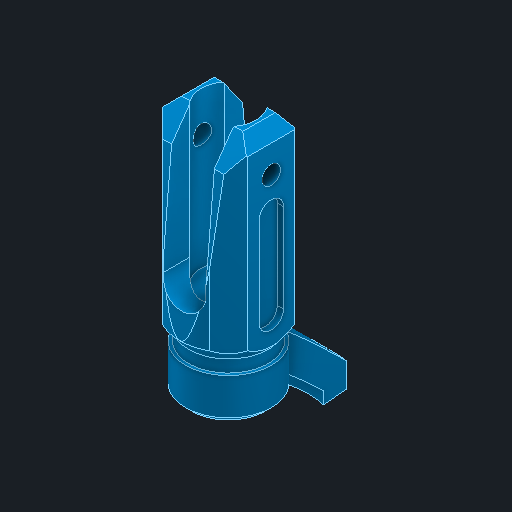
# Autodesk Inventor part: RotorArm
Saved by Autodesk Inventor 2023.2 (Build 272271000, 271)
## iProperties
Created: 2023-03-30
Part Number: RotorArm
Material: Aluminium 6061
Document SubType Name: Modeling
Designer: tadeu
Density: 2.7 g/cm^3
Appearance: Aluminium - flach
Author: tadeu
Autodesk Inventor part; units mm, degrees
ref_plane "YZ Plane" through (0, 0, 0) normal (1, 0, 0) x (0, 1, 0)
ref_plane "XZ Plane" through (0, 0, 0) normal (0, 1, 0) x (-1, 0, 0)
ref_plane "XY Plane" through (0, 0, 0) normal (0, 0, 1) x (1, 0, 0)
sketch "Skizze1" plane through (0, 0, 0) normal (0, 1, 0) x (-1, 0, 0)
  circle A0 centre (0, 0) radius 7
  circle A1 centre (0, 0) radius 6.5
  circle A2 centre (0, 0) radius 2
  dimension "d0" = 14
  dimension "d3" = 13
  dimension "d54" = 4
  constraints: 3 centre point, 3 coincident
  measures "d0" diameter of A0
  measures "d3" diameter of A1
  measures "d54" diameter of A2
extrude "Extrusion1" add sketch "Skizze1" against normal blind 7 contours A0 | A1 | A2
chamfer "Fase1" distance 1 angle 45 1 edges at (7, -7, 0)
extrude "Extrusion2" add sketch "Skizze1" along normal blind 4 contours A1 | A2
sketch "Skizze2" plane through (0, 4, 0) normal (0, 1, 0) x (1, 0, 0)
  circle A0 centre (0, 0) radius 8
  dimension "d9" = 16
  constraints: 1 centre point, 1 coincident
  measures "d9" diameter of A0
extrude "Extrusion3" add sketch "Skizze2" along normal blind 29.5
extrude "Extrusion7" cut sketch "Skizze1" along normal through all both and the other way through all contours A2
chamfer "Fase2" distance 1.5 distance2 2 1 edges at (6.5, 4, 0) measured on face at (7, 4, 0)
sketch "Skizze3" plane through (0, 33.5, 0) normal (0, 1, 0) x (1, 0, 0)
  circle A0 centre (0, 0) radius 8 projected
  line L0 (-7, 3.873) -> (-7, -3.873)
  line L1 (7, -3.873) -> (7, 3.873)
  line L2 (7, 3.873) -> (-7, -3.873) construction
  line L3 (-7, 3.873) -> (7, -3.873) construction
  arc A1 (7, -3.873) -> (7, 3.873) centre (0, 0) ccw
  arc A2 (-7, 3.873) -> (-7, -3.873) centre (0, 0) ccw
  line L4 (7, -3.873) -> (3.873, -7)
  arc A3 (3.873, -7) -> (7, -3.873) centre (0, 0) ccw
  line L5 (7, 3.873) -> (3.873, 7)
  arc A4 (7, 3.873) -> (3.873, 7) centre (0, 0) ccw
  line L6 (0, -7.9724) -> (0, 9.2995) construction
  line L7 (-7, -3.873) -> (-3.873, -7)
  line L8 (-7, -3.873) -> (-3.873, -7)
  line L9 (-7, 3.873) -> (-3.873, 7)
  arc A5 (-3.873, -7) -> (-7, -3.873) centre (0, 0) ccw
  arc A6 (-7, -3.873) -> (-3.873, -7) centre (0, 0) ccw
  arc A7 (-3.873, 7) -> (-7, 3.873) centre (0, 0) ccw
  line L10 (0, 14.4823) -> (0, -23.1738) construction
  point P0 (-4.6045, -6.2685)
  point P1 (-7, 3.873)
  point P2 (-7, 3.873)
  point P3 (6.046, 5.2389)
  point P4 (7, -3.873)
  point P5 (7, -3.873)
  dimension "d15" = 14
  dimension "d26" = 7
  dimension "d33" = 135
  dimension "d34" = 135
  dimension "d35" = 135
  dimension "d36" = 135
  dimension "d48" = 7
  dimension "d49" = 14
  constraints: 22 end point, 16 point on circle, 7 centre point, 2 midpoint, 2 parallel, 2 point on line, 2 vertical, 1 concentric, 13 other
  measures "d15" distance of L1.start L0.end
  measures "d26" distance between parallel lines of L0 L10
  measures "d33" angle of L0 L9
  measures "d34" angle of L7 L0
  measures "d35" angle of L1 L5
  measures "d36" angle of L4 L1
  measures "d48" distance from line of L10 L1.end
  measures "d49" diameter of L0.start L6
extrude "Extrusion4" cut sketch "Skizze3" against normal through all contours A0 L1 | L5 A0 | A0 L4 | L9 A0 | A0 L7 | L0 A0
sketch "Skizze5" plane through (0, 0, 0) normal (0, 0, 1) x (1, 0, 0)
  line L0 (-3.5, 11.5) -> (-3.5, 33.5)
  line L1 (3.873, 33.5) -> (-3.873, 33.5) projected
  line L2 (-7, 33.5) -> (-3.873, 33.5) projected
  line L3 (6.5, 2) -> (-6.5, 2) projected
  line L4 (3.5, 11.5) -> (3.5, 33.5)
  line L5 (-3.5, 33.5) -> (3.5, 33.5)
  line L6 (7, 33.5) -> (3.873, 33.5) projected
  arc A0 (-3.5, 11.5) -> (3.5, 11.5) centre (0, 11.5) ccw
  line L7 (-3.873, 33.5) -> (-3.873, 4) projected
  line L8 (-7, 4) -> (-7, 33.5) projected
  point P0 (0, 0)
  dimension "d28" = 22
  dimension "d29" = 9.5
  dimension "d51" = 7
  constraints: 6 end point, 2 point on circle, 1 centre point, 1 collinear, 1 point on line, 1 vertical
  measures "d28" distance from line of L1 A0.centre
  measures "d29" distance from line of L3 A0.centre
  measures "d51" distance from line of L8 A0.centre
extrude "Extrusion5" cut sketch "Skizze5" along normal through all both and the other way through all
sketch "Skizze6" plane through (0, 0, 0) normal (1, 0, 0) x (0, 1, 0)
  line L0 (4, -8) -> (8, -8) projected
  line L1 (4, -8) -> (29, -5.8128)
  line L2 (4, 8) -> (8, 8) projected
  line L3 (4, -8) -> (4, -7) projected
  line L4 (44.5462, 8) -> (44.5462, -8)
  line L5 (8, -8) -> (44.5462, -8)
  line L6 (8, -8) -> (4, -8)
  line L7 (4, 8) -> (8, 8)
  line L8 (4, 8) -> (29, 5.8128)
  line L9 (4, 8) -> (29.0955, 8) construction
  line L10 (4, 7) -> (4, 8) projected
  line L11 (29, -5.8128) -> (37.3015, 0)
  line L12 (29, -5.8128) -> (39.1343, -5.8128) construction
  line L13 (29, 5.8128) -> (37.3015, 0)
  line L14 (29, 5.8128) -> (39.1343, 5.8128) construction
  line L15 (44.5462, 8) -> (4, 8)
  point P0 (0, 0)
  dimension "d39" = 25
  dimension "d42" = 5
  dimension "d43" = 25
  dimension "d44" = 5
  dimension "d52" = 35
  dimension "d53" = 35
  constraints: 24 end point, 4 horizontal, 3 equal length, 1 collinear, 1 perpendicular, 1 point on line, 1 vertical
  measures "d39" distance from line of L3 L1.end
  measures "d42" angle of L8 L9
  measures "d43" distance from line of L10 L8.end
  measures "d44" angle of L5 L1
  measures "d52" angle of L12 L11
  measures "d53" angle of L13 L14
extrude "Extrusion6" cut sketch "Skizze6" along normal through all both and the other way through all
sketch "Skizze11" plane through (0, 0, 0) normal (1, 0, 0) x (0, 1, 0)
  line L0 (0, -7) -> (-10, -17)
  line L1 (0, -7) -> (21.0348, -7) construction
  line L2 (-6, -7) -> (-12, -13)
  line L3 (-12, -13) -> (-14, -13)
  line L4 (-10, -17) -> (-14, -17)
  line L5 (-14, -13) -> (-14, -17)
  line L6 (42.8428, 0) -> (-25, 0)
  line L7 (0, -7) -> (-6, -7)
  point P0 (0, 0)
  dimension "d64" = 135
  dimension "d67" = 2
  constraints: 16 end point, 4 horizontal, 1 parallel, 1 vertical
  measures "d64" angle of L0 L1
  measures "d67" distance of L2.end L3.end
revolve "Umdrehung2" add sketch "Skizze11" angle 90 mid plane about axis through (0, 42.8428, 0) along (0, -1, 0)
sketch "Skizze16" plane through (0, -7, 0) normal (0, -1, 0) x (1, 0, 0)
  line L0 (0, 0) -> (0, -8.9764) construction
  arc A0 (-4.9497, -4.9497) -> (4.9497, -4.9497) centre (0, 0) ccw construction
  line L1 (12.0208, -12.0208) -> (4.9497, -4.9497) projected
  arc A1 (3.5, -6.0622) -> (4.9497, -4.9497) centre (0, 0) ccw
  arc A2 (2.5, -16.8152) -> (12.0208, -12.0208) centre (0, 0) ccw
  line L2 (2.5, -16.8152) -> (3.5, -6.0622)
  line L3 (9.1924, -9.1924) -> (12.0208, -12.0208) projected
  line L4 (4.9497, -4.9497) -> (12.0208, -12.0208)
  line L5 (-12.0208, -12.0208) -> (-4.9497, -4.9497)
  arc A3 (-4.9497, -4.9497) -> (-3.5, -6.0622) centre (0, 0) ccw
  arc A4 (-12.0208, -12.0208) -> (-2.5, -16.8152) centre (0, 0) ccw
  line L6 (-2.5, -16.8152) -> (-3.5, -6.0622)
  line L7 (-9.1924, -9.1924) -> (-12.0208, -12.0208)
  line L8 (-4.9497, -4.9497) -> (-12.0208, -12.0208)
  dimension "d79" = 3.5
  dimension "d80" = 2.5
  constraints: 14 end point, 9 point on circle, 7 symmetric about line, 4 centre point, 1 collinear, 1 vertical, 2 other
  measures "d79" distance from line of L0 L2.end
  measures "d80" distance from line of L0 L2.start
extrude "Extrusion12" cut sketch "Skizze16" along normal mid plane 14
chamfer "Fase4" distance 2 angle 45 2 edges at (7, 33.5, 0) (-7, 33.5, 0)
sketch "Skizze17" plane through (7, 4, 3.873) normal (1, 0, 0) x (0, 0, -1)
  line L0 (7.746, 0) -> (7.746, 27.5) projected
  line L1 (0, 0) -> (0, 27.5) projected
  line L2 (0, 27.5) -> (7.746, 27.5) projected
  line L3 (10.873, 11.4301) -> (10.873, 0) projected
  line L4 (-3.127, 0) -> (-3.127, 11.4301) projected
  line L5 (6.5348, 29.5) -> (1.2111, 29.5) projected
  point P0 (3.873, -4)
  point P1 (3.873, 23)
  dimension "d100" = 4.5
  dimension "d101" = 7
  dimension "d102" = 14
  dimension "d122" = 2
  measures "d100" distance from line of L2 point (3.873, 23)
  measures "d101" distance from line of point (3.873, 23) L3
  measures "d102" distance between parallel lines of L4 L3
  measures "d122" distance between parallel lines of L5 L2
hole "Bohrung1" at (7, 27, 0) direction (-1, 0, 0) diameter 3 end through all
sketch "Skizze18" plane through (7, 4, 3.873) normal (1, 0, 0) x (0, 0, -1)
  arc A0 (5.873, 17.5) -> (1.873, 17.5) centre (3.873, 17.5) ccw
  line L0 (10.873, 11.4301) -> (10.873, 0) projected
  line L1 (0, 27.5) -> (7.746, 27.5) projected
  arc A1 (1.873, 3) -> (5.873, 3) centre (3.873, 3) ccw
  line L2 (5.873, 17.5) -> (5.873, 3)
  line L3 (1.873, 17.5) -> (1.873, 3)
  point P0 (3.873, -4)
  dimension "d103" = 4
  dimension "d104" = 7
  dimension "d105" = 10
  dimension "d106" = 4
  dimension "d107" = 14.5
  constraints: 4 end point, 4 point on circle, 2 centre point
  measures "d103" diameter of A0
  measures "d104" distance from line of L0 A0.centre
  measures "d105" distance from line of L1 A0.centre
  measures "d106" diameter of A1
  measures "d107" distance of A1.centre A0.centre
extrude "Extrusion13" cut sketch "Skizze18" against normal blind 1
mirror "Spiegeln1" about plane through (0, 0, 0) normal (1, 0, 0) of "Extrusion13"
sketch "Skizze19" plane through (0, -14, 0) normal (0, -1, 0) x (1, 0, 0)
  arc A0 (-2.8849, -12.6758) -> (2.8849, -12.6758) centre (0, 0) ccw projected
  line L0 (0, 0) -> (0, -25.3641) construction
  point P0 (0, 0)
  point P1 (0, -15)
  dimension "d117" = 15
  dimension "d118" = 0
  constraints: 2 end point, 1 vertical
  measures "d117" distance of point (0, -15) L0.start
  measures "d118" distance from line of L0 point (0, -15)
hole "Bohrung2" at (0, -14, -15) direction (0, 1, 0) diameter 2 end through all
sketch "Skizze20" plane through (0, 33.5, 0) normal (0, 1, 0) x (1, 0, 0)
  circle A0 centre (0, 0) radius 4.5
  dimension "d119" = 9
  constraints: 1 centre point, 1 coincident
  measures "d119" diameter of A0
extrude "Extrusion14" cut sketch "Skizze20" against normal blind 25.5
